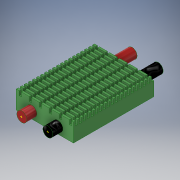
# Autodesk Inventor part: Power Switch
Saved by Autodesk Inventor 2019.2 (Build 232265000, 265)
## iProperties
Created: 2018-12-12
Part Number: Power Switch
Material: Generic
Document SubType Name: Modeling
Designer: Petar
Density: 1 g/cm^3
Appearance: Smooth - Dark Forest Green
Author: Petar
Autodesk Inventor part; units mm, degrees
ref_plane "YZ Plane" through (0, 0, 0) normal (1, 0, 0) x (0, 1, 0)
ref_plane "XZ Plane" through (0, 0, 0) normal (0, 1, 0) x (-1, 0, 0)
ref_plane "XY Plane" through (0, 0, 0) normal (0, 0, 1) x (1, 0, 0)
sketch "Sketch1" plane through (0, 0, 0) normal (0, 1, 0) x (-1, 0, 0)
  line L0 (8.035, 1.5055) -> (-20.465, 1.5055)
  line L1 (-20.465, 1.5055) -> (-20.465, 41.5055)
  line L2 (-20.465, 41.5055) -> (8.035, 41.5055)
  line L3 (8.035, 41.5055) -> (8.035, 1.5055)
  line L4 (-6.215, 41.5055) -> (-6.215, 1.5055) construction
  point P0 (0, 0)
  dimension "d0" = 28.5
  dimension "d1" = 40
  constraints: 10 end point, 2 midpoint, 2 parallel, 1 horizontal, 1 perpendicular
  measures "d0" distance of L1.end L2.end
  measures "d1" distance of L0.end L1.end
extrude "Extrusion1" add sketch "Sketch1" along normal blind 9.1
sketch "Sketch2" plane through (20.465, 0, 41.5055) normal (1, 0, 0) x (0, 0, -1)
  line L0 (0, 0) -> (0, 9.1) projected
  line L1 (40, 9.1) -> (0, 9.1) projected
  line L2 (1, 9.1) -> (2, 9.1)
  line L3 (2, 9.1) -> (2, 7)
  line L4 (2, 7) -> (1, 7)
  line L5 (1, 7) -> (1, 9.1)
  point P0 (41.5055, 0)
  dimension "d4" = 1
  constraints: 8 end point, 2 parallel, 1 horizontal, 1 perpendicular, 1 point on line
  measures "d4" distance between parallel lines of L0 L5
sketch "Sketch3" plane through (-8.035, 0, 41.5055) normal (0, 0, 1) x (1, 0, 0)
  line L0 (28.5, 0) -> (28.5, 9.1) projected
  line L1 (28.5, 9.1) -> (0, 9.1) projected
  line L2 (27.5, 9.1) -> (26.5, 9.1)
  line L3 (26.5, 9.1) -> (26.5, 7)
  line L4 (26.5, 7) -> (27.5, 7)
  line L5 (27.5, 7) -> (27.5, 9.1)
  point P0 (8.035, 0)
  dimension "d5" = 1
  dimension "d6" = 1
  constraints: 8 end point, 2 parallel, 1 horizontal, 1 perpendicular, 1 point on line
  measures "d5" distance of L4.end L3.end
  measures "d6" distance between parallel lines of L0 L5
extrude "Extrusion2" cut sketch "Sketch3" against normal through all
pattern_linear "Rectangular Pattern1" count 6 spacing 5 along (-1, 0, 0) of "Extrusion2"
extrude "Extrusion3" cut sketch "Sketch2" against normal through all
pattern_linear "Rectangular Pattern2" count 20 spacing 2 along (0, 0, -1) of "Extrusion3"
sketch "Sketch4" plane through (0, 0, 0) normal (0, -1, 0) x (1, 0, 0)
  line L0 (-8.035, 1.5055) -> (20.465, 1.5055) projected
  line L1 (20.465, 41.5055) -> (-8.035, 41.5055) projected
  line L2 (-6.4407, 25.3147) -> (18.8707, 25.3147) construction
  line L3 (18.8707, 25.3147) -> (18.8707, 17.0738) construction
  line L4 (18.8707, 17.0738) -> (-6.4407, 17.0738) construction
  line L5 (-6.4407, 17.0738) -> (-6.4407, 25.3147) construction
  line L6 (6.215, 1.5055) -> (6.215, 41.5055) construction
  line L7 (-3.9344, 22.3432) -> (-3.9344, 26.3432)
  line L8 (-3.9344, 26.3432) -> (-2.6386, 26.3432)
  spline S0 degree 2 poles (-2.6386, 26.3432) (-1.9008, 26.3432) (-1.6783, 26.2822) knots 0 0 0 1 1 1
  spline S1 degree 2 poles (-1.6783, 26.2822) (-1.3337, 26.1938) (-0.8703, 25.5901) (-0.8703, 25.1115) knots 0 0 0 1 2 2 2
  spline S2 degree 2 poles (-0.8703, 25.1115) (-0.8703, 24.7456) (-1.1386, 24.2426) (-1.5502, 23.956) (-1.7636, 23.9102) knots 0 0 0 1 2 3 3 3
  spline S3 degree 2 poles (-1.7636, 23.9102) (-2.0502, 23.8523) (-2.599, 23.8523) knots 0 0 0 1 1 1
  line L9 (-2.599, 23.8523) -> (-3.1264, 23.8523)
  line L10 (-3.1264, 23.8523) -> (-3.1264, 22.3432)
  line L11 (-3.1264, 22.3432) -> (-3.9344, 22.3432)
  line L12 (-3.1264, 25.6663) -> (-3.1264, 24.5291)
  line L13 (-3.1264, 24.5291) -> (-2.6844, 24.5291)
  spline S4 degree 2 poles (-2.6844, 24.5291) (-2.2057, 24.5291) (-1.8856, 24.6541) (-1.7026, 24.9224) (-1.7026, 25.0993) knots 0 0 0 1 2 3 3 3
  spline S5 degree 2 poles (-1.7026, 25.0993) (-1.7026, 25.3188) (-1.9587, 25.6023) (-2.1569, 25.6389) knots 0 0 0 1 2 2 2
  spline S6 degree 2 poles (-2.1569, 25.6389) (-2.3002, 25.6663) (-2.7362, 25.6663) knots 0 0 0 1 1 1
  line L14 (-2.7362, 25.6663) -> (-3.1264, 25.6663)
  spline S7 degree 2 poles (-0.3703, 24.3188) (-0.3703, 24.9285) (-0.1874, 25.3432) knots 0 0 0 1 1 1
  spline S8 degree 2 poles (-0.1874, 25.3432) (-0.0502, 25.6481) (0.4224, 26.1359) (0.7028, 26.2517) knots 0 0 0 1 2 2 2
  spline S9 degree 2 poles (0.7028, 26.2517) (1.0748, 26.4102) (1.5656, 26.4102) knots 0 0 0 1 1 1
  spline S10 degree 2 poles (1.5656, 26.4102) (2.4498, 26.4102) (3.5108, 25.3127) (3.5108, 24.3371) knots 0 0 0 1 2 2 2
  spline S11 degree 2 poles (3.5108, 24.3371) (3.5108, 23.3706) (2.4559, 22.2761) (1.5748, 22.2761) knots 0 0 0 1 2 2 2
  spline S12 degree 2 poles (1.5748, 22.2761) (0.6845, 22.2761) (-0.3703, 23.3645) (-0.3703, 24.3188) knots 0 0 0 1 2 2 2
  spline S13 degree 2 poles (0.462, 24.3462) (0.462, 23.6663) (1.09, 22.9651) (1.5748, 22.9651) knots 0 0 0 1 2 2 2
  spline S14 degree 2 poles (1.5748, 22.9651) (2.0595, 22.9651) (2.6785, 23.6602) (2.6785, 24.3554) knots 0 0 0 1 2 2 2
  spline S15 degree 2 poles (2.6785, 24.3554) (2.6785, 25.0444) (2.0748, 25.7212) (1.5748, 25.7212) knots 0 0 0 1 2 2 2
  spline S16 degree 2 poles (1.5748, 25.7212) (1.0748, 25.7212) (0.462, 25.0352) (0.462, 24.3462) knots 0 0 0 1 2 2 2
  line L15 (4.6998, 22.3432) -> (3.7516, 26.3432)
  line L16 (3.7516, 26.3432) -> (4.5809, 26.3432)
  line L17 (4.5809, 26.3432) -> (5.1815, 23.5962)
  line L18 (5.1815, 23.5962) -> (5.9102, 26.3432)
  line L19 (5.9102, 26.3432) -> (6.8705, 26.3432)
  line L20 (6.8705, 26.3432) -> (7.5748, 23.5505)
  line L21 (7.5748, 23.5505) -> (8.1876, 26.3432)
  line L22 (8.1876, 26.3432) -> (9.0016, 26.3432)
  line L23 (9.0016, 26.3432) -> (8.0291, 22.3432)
  line L24 (8.0291, 22.3432) -> (7.1693, 22.3432)
  line L25 (7.1693, 22.3432) -> (6.3766, 25.334)
  line L26 (6.3766, 25.334) -> (5.5809, 22.3432)
  line L27 (5.5809, 22.3432) -> (4.6998, 22.3432)
  line L28 (9.4163, 22.3432) -> (9.4163, 26.3432)
  line L29 (9.4163, 26.3432) -> (12.3827, 26.3432)
  line L30 (12.3827, 26.3432) -> (12.3827, 25.6663)
  line L31 (12.3827, 25.6663) -> (10.2242, 25.6663)
  line L32 (10.2242, 25.6663) -> (10.2242, 24.7791)
  line L33 (10.2242, 24.7791) -> (12.2333, 24.7791)
  line L34 (12.2333, 24.7791) -> (12.2333, 24.1023)
  line L35 (12.2333, 24.1023) -> (10.2242, 24.1023)
  line L36 (10.2242, 24.1023) -> (10.2242, 23.02)
  line L37 (10.2242, 23.02) -> (12.4589, 23.02)
  line L38 (12.4589, 23.02) -> (12.4589, 22.3432)
  line L39 (12.4589, 22.3432) -> (9.4163, 22.3432)
  line L40 (13.1449, 22.3432) -> (13.1449, 26.3432)
  line L41 (13.1449, 26.3432) -> (14.8461, 26.3432)
  spline S17 degree 2 poles (14.8461, 26.3432) (15.4894, 26.3432) (16.0687, 26.1267) (16.4193, 25.5779) (16.4193, 25.2212) knots 0 0 0 1 2 3 3 3
  spline S18 degree 2 poles (16.4193, 25.2212) (16.4193, 24.7731) (15.8919, 24.1846) (15.3644, 24.1084) knots 0 0 0 1 2 2 2
  spline S19 degree 2 poles (15.3644, 24.1084) (15.6266, 23.956) (15.9681, 23.5901) (16.2577, 23.1237) knots 0 0 0 1 2 2 2
  line L42 (16.2577, 23.1237) -> (16.7455, 22.3432)
  line L43 (16.7455, 22.3432) -> (15.7791, 22.3432)
  line L44 (15.7791, 22.3432) -> (15.1967, 23.2151)
  spline S20 degree 2 poles (15.1967, 23.2151) (14.8827, 23.6816) (14.6541, 23.9255) (14.398, 24.0139) (14.1175, 24.0139) knots 0 0 0 1 2 3 3 3
  line L45 (14.1175, 24.0139) -> (13.9528, 24.0139)
  line L46 (13.9528, 24.0139) -> (13.9528, 22.3432)
  line L47 (13.9528, 22.3432) -> (13.1449, 22.3432)
  line L48 (13.9528, 24.6511) -> (14.5504, 24.6511)
  spline S21 degree 2 poles (14.5504, 24.6511) (15.1327, 24.6511) (15.4224, 24.7487) (15.587, 24.9895) (15.587, 25.1694) knots 0 0 0 1 2 3 3 3
  spline S22 degree 2 poles (15.587, 25.1694) (15.587, 25.3706) (15.3705, 25.6206) (15.1754, 25.6541) knots 0 0 0 1 2 2 2
  spline S23 degree 2 poles (15.1754, 25.6541) (15.0748, 25.6663) (14.5839, 25.6663) knots 0 0 0 1 1 1
  line L49 (14.5839, 25.6663) -> (13.9528, 25.6663)
  line L50 (13.9528, 25.6663) -> (13.9528, 24.6511)
  line L51 (-4.6051, 17.3532) -> (-3.8185, 17.4295)
  spline S24 degree 2 poles (-3.8185, 17.4295) (-3.7484, 17.0331) (-3.3124, 16.6612) (-2.9465, 16.6612) knots 0 0 0 1 2 2 2
  spline S25 degree 2 poles (-2.9465, 16.6612) (-2.5563, 16.6612) (-2.16, 16.9904) (-2.16, 17.213) knots 0 0 0 1 2 2 2
  spline S26 degree 2 poles (-2.16, 17.213) (-2.16, 17.3563) (-2.3276, 17.5545) (-2.535, 17.6276) knots 0 0 0 1 2 2 2
  spline S27 degree 2 poles (-2.535, 17.6276) (-2.6752, 17.6764) (-3.1813, 17.8014) knots 0 0 0 1 1 1
  spline S28 degree 2 poles (-3.1813, 17.8014) (-3.8307, 17.963) (-4.0929, 18.1978) knots 0 0 0 1 1 1
  spline S29 degree 2 poles (-4.0929, 18.1978) (-4.4618, 18.527) (-4.4618, 18.9996) knots 0 0 0 1 1 1
  spline S30 degree 2 poles (-4.4618, 18.9996) (-4.4618, 19.3075) (-4.1142, 19.838) (-3.4618, 20.1154) (-3.0014, 20.1154) knots 0 0 0 1 2 3 3 3
  spline S31 degree 2 poles (-3.0014, 20.1154) (-2.2484, 20.1154) (-1.4862, 19.4569) (-1.4679, 18.9051) knots 0 0 0 1 2 2 2
  line L52 (-1.4679, 18.9051) -> (-2.2758, 18.8685)
  spline S32 degree 2 poles (-2.2758, 18.8685) (-2.3276, 19.1764) (-2.6691, 19.4478) (-3.0106, 19.4478) knots 0 0 0 1 2 2 2
  spline S33 degree 2 poles (-3.0106, 19.4478) (-3.3642, 19.4478) (-3.5624, 19.3045) knots 0 0 0 1 1 1
  spline S34 degree 2 poles (-3.5624, 19.3045) (-3.6905, 19.2099) (-3.6905, 19.0545) knots 0 0 0 1 1 1
  spline S35 degree 2 poles (-3.6905, 19.0545) (-3.6905, 18.9142) (-3.5715, 18.8106) knots 0 0 0 1 1 1
  spline S36 degree 2 poles (-3.5715, 18.8106) (-3.4161, 18.6825) (-2.2362, 18.4051) (-1.6722, 18.1093) (-1.352, 17.5941) (-1.352, 17.213) knots 0 0 0 1 2 3 4 4 4
  spline S37 degree 2 poles (-1.352, 17.213) (-1.352, 16.8715) (-1.7331, 16.2709) (-2.4313, 15.9782) (-2.9526, 15.9782) knots 0 0 0 1 2 3 3 3
  spline S38 degree 2 poles (-2.9526, 15.9782) (-3.7118, 15.9782) (-4.5258, 16.6795) (-4.6051, 17.3532) knots 0 0 0 1 2 2 2
  line L53 (-0.1112, 16.0484) -> (-1.0594, 20.0484)
  line L54 (-1.0594, 20.0484) -> (-0.2301, 20.0484)
  line L55 (-0.2301, 20.0484) -> (0.3705, 17.3014)
  line L56 (0.3705, 17.3014) -> (1.0992, 20.0484)
  line L57 (1.0992, 20.0484) -> (2.0595, 20.0484)
  line L58 (2.0595, 20.0484) -> (2.7638, 17.2557)
  line L59 (2.7638, 17.2557) -> (3.3766, 20.0484)
  line L60 (3.3766, 20.0484) -> (4.1906, 20.0484)
  line L61 (4.1906, 20.0484) -> (3.2181, 16.0484)
  line L62 (3.2181, 16.0484) -> (2.3583, 16.0484)
  line L63 (2.3583, 16.0484) -> (1.5656, 19.0392)
  line L64 (1.5656, 19.0392) -> (0.7699, 16.0484)
  line L65 (0.7699, 16.0484) -> (-0.1112, 16.0484)
  line L66 (4.5778, 16.0484) -> (4.5778, 20.0484)
  line L67 (4.5778, 20.0484) -> (5.3858, 20.0484)
  line L68 (5.3858, 20.0484) -> (5.3858, 16.0484)
  line L69 (5.3858, 16.0484) -> (4.5778, 16.0484)
  line L70 (7.0565, 16.0484) -> (7.0565, 19.3715)
  line L71 (7.0565, 19.3715) -> (5.8705, 19.3715)
  line L72 (5.8705, 19.3715) -> (5.8705, 20.0484)
  line L73 (5.8705, 20.0484) -> (9.0474, 20.0484)
  line L74 (9.0474, 20.0484) -> (9.0474, 19.3715)
  line L75 (9.0474, 19.3715) -> (7.8644, 19.3715)
  line L76 (7.8644, 19.3715) -> (7.8644, 16.0484)
  line L77 (7.8644, 16.0484) -> (7.0565, 16.0484)
  line L78 (12.1297, 17.5209) -> (12.9132, 17.274)
  spline S39 degree 2 poles (12.9132, 17.274) (12.7333, 16.6185) (11.8949, 15.9813) (11.2516, 15.9813) knots 0 0 0 1 2 2 2
  spline S40 degree 2 poles (11.2516, 15.9813) (10.4559, 15.9813) (9.4285, 17.0697) (9.4285, 18.0118) knots 0 0 0 1 2 2 2
  spline S41 degree 2 poles (9.4285, 18.0118) (9.4285, 19.0118) (10.4589, 20.1154) (11.3004, 20.1154) knots 0 0 0 1 2 2 2
  spline S42 degree 2 poles (11.3004, 20.1154) (12.0321, 20.1154) (12.4925, 19.6825) knots 0 0 0 1 1 1
  spline S43 degree 2 poles (12.4925, 19.6825) (12.7638, 19.4264) (12.901, 18.9478) knots 0 0 0 1 1 1
  line L79 (12.901, 18.9478) -> (12.1022, 18.7557)
  spline S44 degree 2 poles (12.1022, 18.7557) (12.0321, 19.0667) (11.5809, 19.4264) (11.2608, 19.4264) knots 0 0 0 1 2 2 2
  spline S45 degree 2 poles (11.2608, 19.4264) (10.8156, 19.4264) (10.2608, 18.7892) (10.2608, 18.0728) knots 0 0 0 1 2 2 2
  spline S46 degree 2 poles (10.2608, 18.0728) (10.2608, 17.3136) (10.8065, 16.6703) (11.2425, 16.6703) knots 0 0 0 1 2 2 2
  spline S47 degree 2 poles (11.2425, 16.6703) (11.5656, 16.6703) (12.0291, 17.0819) (12.1297, 17.5209) knots 0 0 0 1 2 2 2
  line L80 (13.6083, 16.0484) -> (13.6083, 20.0484)
  line L81 (13.6083, 20.0484) -> (14.4163, 20.0484)
  line L82 (14.4163, 20.0484) -> (14.4163, 18.4752)
  line L83 (14.4163, 18.4752) -> (15.9986, 18.4752)
  line L84 (15.9986, 18.4752) -> (15.9986, 20.0484)
  line L85 (15.9986, 20.0484) -> (16.8065, 20.0484)
  line L86 (16.8065, 20.0484) -> (16.8065, 16.0484)
  line L87 (16.8065, 16.0484) -> (15.9986, 16.0484)
  line L88 (15.9986, 16.0484) -> (15.9986, 17.7984)
  line L89 (15.9986, 17.7984) -> (14.4163, 17.7984)
  line L90 (14.4163, 17.7984) -> (14.4163, 16.0484)
  line L91 (14.4163, 16.0484) -> (13.6083, 16.0484)
  point P0 (0, 0)
  constraints: 2 end point, 2 midpoint, 3 other
emboss "Emboss1" sketch "Sketch4" operation cut depth 0.1 direction (0, 1, 0)
sketch "Sketch5" plane through (20.465, 0, 1.5055) normal (0, 0, -1) x (-1, 0, 0)
  line L0 (28.5, 7) -> (0, 7) projected
  line L1 (28.5, 0) -> (0, 0) projected
  circle A0 centre (20.75, 3.5) radius 2.5
  line L2 (14.25, 0) -> (14.25, 7) construction
  circle A1 centre (7.75, 3.5) radius 2.5
  point P0 (20.465, 0)
  dimension "d19" = 5
  dimension "d20" = 6.5
  constraints: 2 centre point, 2 end point, 2 midpoint, 1 symmetric about line, 1 other
  measures "d19" diameter of A0
  measures "d20" distance from line of L2 A0.centre
extrude "Extrusion4" add sketch "Sketch5" along normal blind 10
sketch "Sketch6" plane through (-8.035, 0, 41.5055) normal (0, 0, 1) x (1, 0, 0)
  circle A0 centre (20.75, 3.5) radius 2.5 projected
  circle A1 centre (20.75, 3.5) radius 2.5 projected
  circle A2 centre (7.75, 3.5) radius 2.5 projected
  circle A3 centre (7.75, 3.5) radius 2.5 projected
  point P0 (8.035, 0)
extrude "Extrusion5" add sketch "Sketch6" along normal blind 5
sketch "Sketch7" plane through (12.715, 3.5, 46.5055) normal (0, 0, 1) x (1, 0, 0)
  circle A0 centre (0, 0) radius 2.5 projected
sketch "Sketch8" plane through (-0.285, 3.5, 46.5055) normal (0, 0, 1) x (1, 0, 0)
  circle A0 centre (0, 0) radius 2.5 projected
sketch "Sketch9" plane through (-0.285, 3.5, -8.4945) normal (0, 0, -1) x (-1, 0, 0)
  circle A0 centre (0, 0) radius 2.5 projected
sketch "Sketch10" plane through (12.715, 3.5, -8.4945) normal (0, 0, -1) x (-1, 0, 0)
  circle A0 centre (0, 0) radius 2.5 projected
sketch "Sketch11" plane through (0, 0, 0) normal (0, -1, 0) x (1, 0, 0)
  line L0 (20.465, 1.5055) -> (20.465, 41.5055) projected
  line L1 (-8.035, 41.5055) -> (-8.035, 1.5055) projected
  line L2 (18.5791, 2.1286) -> (18.5791, 10.0514) construction
  line L3 (18.5791, 10.0514) -> (19.6923, 10.0514) construction
  line L4 (19.6923, 10.0514) -> (19.6923, 2.1286) construction
  line L5 (19.6923, 2.1286) -> (18.5791, 2.1286) construction
  line L6 (20.465, 21.5055) -> (-8.035, 21.5055) construction
  line L7 (19.0462, 3.0806) -> (19.425, 2.2873)
  line L8 (19.425, 2.2873) -> (19.294, 2.2873)
  line L9 (19.294, 2.2873) -> (19.0016, 2.9023)
  line L10 (19.0016, 2.9023) -> (18.7101, 2.2873)
  line L11 (18.7101, 2.2873) -> (18.5791, 2.2873)
  line L12 (18.5791, 2.2873) -> (18.9579, 3.0806)
  line L13 (18.9579, 3.0806) -> (19.0462, 3.0806)
  line L14 (19.0462, 4.1815) -> (19.425, 3.3882)
  line L15 (19.425, 3.3882) -> (19.294, 3.3882)
  line L16 (19.294, 3.3882) -> (19.0016, 4.0032)
  line L17 (19.0016, 4.0032) -> (18.7101, 3.3882)
  line L18 (18.7101, 3.3882) -> (18.5791, 3.3882)
  line L19 (18.5791, 3.3882) -> (18.9579, 4.1815)
  line L20 (18.9579, 4.1815) -> (19.0462, 4.1815)
  line L21 (19.0462, 5.2824) -> (19.425, 4.489)
  line L22 (19.425, 4.489) -> (19.294, 4.489)
  line L23 (19.294, 4.489) -> (19.0016, 5.1041)
  line L24 (19.0016, 5.1041) -> (18.7101, 4.489)
  line L25 (18.7101, 4.489) -> (18.5791, 4.489)
  line L26 (18.5791, 4.489) -> (18.9579, 5.2824)
  line L27 (18.9579, 5.2824) -> (19.0462, 5.2824)
  line L28 (19.0462, 6.3833) -> (19.425, 5.5899)
  line L29 (19.425, 5.5899) -> (19.294, 5.5899)
  line L30 (19.294, 5.5899) -> (19.0016, 6.205)
  line L31 (19.0016, 6.205) -> (18.7101, 5.5899)
  line L32 (18.7101, 5.5899) -> (18.5791, 5.5899)
  line L33 (18.5791, 5.5899) -> (18.9579, 6.3833)
  line L34 (18.9579, 6.3833) -> (19.0462, 6.3833)
  line L35 (19.0462, 7.4842) -> (19.425, 6.6908)
  line L36 (19.425, 6.6908) -> (19.294, 6.6908)
  line L37 (19.294, 6.6908) -> (19.0016, 7.3059)
  line L38 (19.0016, 7.3059) -> (18.7101, 6.6908)
  line L39 (18.7101, 6.6908) -> (18.5791, 6.6908)
  line L40 (18.5791, 6.6908) -> (18.9579, 7.4842)
  line L41 (18.9579, 7.4842) -> (19.0462, 7.4842)
  line L42 (19.0462, 8.5851) -> (19.425, 7.7917)
  line L43 (19.425, 7.7917) -> (19.294, 7.7917)
  line L44 (19.294, 7.7917) -> (19.0016, 8.4068)
  line L45 (19.0016, 8.4068) -> (18.7101, 7.7917)
  line L46 (18.7101, 7.7917) -> (18.5791, 7.7917)
  line L47 (18.5791, 7.7917) -> (18.9579, 8.5851)
  line L48 (18.9579, 8.5851) -> (19.0462, 8.5851)
  line L49 (19.0462, 9.686) -> (19.425, 8.8926)
  line L50 (19.425, 8.8926) -> (19.294, 8.8926)
  line L51 (19.294, 8.8926) -> (19.0016, 9.5077)
  line L52 (19.0016, 9.5077) -> (18.7101, 8.8926)
  line L53 (18.7101, 8.8926) -> (18.5791, 8.8926)
  line L54 (18.5791, 8.8926) -> (18.9579, 9.686)
  line L55 (18.9579, 9.686) -> (19.0462, 9.686)
  point P0 (0, 0)
  constraints: 2 end point, 2 midpoint, 2 other
emboss "Emboss2" sketch "Sketch11" operation cut depth 0.1 direction (0, 1, 0)
sketch "Sketch12" plane through (20.465, 0, 1.5055) normal (0, 0, -1) x (-1, 0, 0)
  line L0 (28.5, 0) -> (0, 0) projected
  line L1 (12, 7) -> (16, 7) projected
  line L2 (14.25, 7) -> (14.25, 0) construction
  circle A0 centre (14.25, 1.1059) radius 0.5
  circle A1 centre (15.75, 1.1059) radius 0.5
  circle A2 centre (12.75, 1.1059) radius 0.5
  point P0 (20.465, 0)
  dimension "d27" = 1
  dimension "d28" = 1
  dimension "d29" = 1.5
  constraints: 3 centre point, 2 end point, 2 point on line, 1 midpoint, 1 symmetric about line, 1 other
  measures "d27" diameter of A0
  measures "d28" diameter of A1
  measures "d29" distance of A0.centre A1.centre
extrude "Extrusion6" add sketch "Sketch12" along normal blind 0.5
fillet "Fillet1" radius 0.5 3 edges at (6.715, 1.1059, 1.0055) (8.215, 1.1059, 1.0055) (5.215, 1.1059, 1.0055)
sketch "Sketch13" plane through (20.465, 0, 1.5055) normal (0, 0, -1) x (-1, 0, 0)
  circle A0 centre (15.75, 1.1059) radius 0.5 projected
sketch "Sketch14" plane through (20.465, 0, 1.5055) normal (0, 0, -1) x (-1, 0, 0)
  circle A0 centre (14.25, 1.1059) radius 0.5 projected
sketch "Sketch15" plane through (20.465, 0, 1.5055) normal (0, 0, -1) x (-1, 0, 0)
  circle A0 centre (12.75, 1.1059) radius 0.5 projected
body "Solid1"
